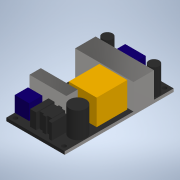
# Autodesk Inventor part: power unit
Saved by Autodesk Inventor 2022 (Build 260153000, 153)
## iProperties
Created: 2024-07-06
Part Number: power unit
Material: Типовые
Document SubType Name: Modeling
Designer: Капустяник Андрей
Density: 1 g/cm^3
Appearance: По умолчанию
Author: Капустяник Андрей
Autodesk Inventor part; units mm, degrees
ref_plane "YZ Plane" through (0, 0, 0) normal (1, 0, 0) x (0, 1, 0)
ref_plane "XZ Plane" through (0, 0, 0) normal (0, 1, 0) x (-1, 0, 0)
ref_plane "XY Plane" through (0, 0, 0) normal (0, 0, 1) x (1, 0, 0)
sketch "Эскиз1" plane through (0, 0, 0) normal (0, 1, 0) x (-1, 0, 0)
  line L0 (-28.51, 53.225) -> (28.51, 53.225)
  line L1 (28.51, 53.225) -> (28.51, -53.225)
  line L2 (28.51, -53.225) -> (-28.51, -53.225)
  line L3 (-28.51, -53.225) -> (-28.51, 53.225)
  line L4 (-28.51, 53.225) -> (28.51, -53.225) construction
  line L5 (28.51, 53.225) -> (-28.51, -53.225) construction
  line L6 (-23.7, 49.095) -> (23.7, 49.095)
  line L7 (23.7, 49.095) -> (23.7, -49.095)
  line L8 (23.7, -49.095) -> (-23.7, -49.095)
  line L9 (-23.7, -49.095) -> (-23.7, 49.095)
  line L10 (-23.7, 49.095) -> (23.7, -49.095) construction
  line L11 (23.7, 49.095) -> (-23.7, -49.095) construction
  circle A0 centre (23.7, 49.095) radius 2
  circle A1 centre (23.7, -49.095) radius 2
  circle A2 centre (-23.7, -49.095) radius 2
  circle A3 centre (-23.7, 49.095) radius 2
  point P0 (0, 0)
  dimension "d0" = 57.02
  dimension "d1" = 106.45
  dimension "d2" = 47.4
  dimension "d3" = 98.19
  dimension "d4" = 4
  dimension "d5" = 4
  dimension "d6" = 4
  dimension "d7" = 4
  constraints: 24 end point, 4 centre point, 4 coincident, 4 midpoint, 4 parallel, 2 horizontal, 2 perpendicular
  measures "d0" distance of L1.end L2.end
  measures "d1" distance of L0.end L1.end
  measures "d2" distance of L7.end L8.end
  measures "d3" distance of L6.end L7.end
  measures "d4" diameter of A0
  measures "d5" diameter of A1
  measures "d6" diameter of A2
  measures "d7" diameter of A3
extrude "Выдавливание1" add sketch "Эскиз1" along normal blind 28 contours L0 L1 L2 L3 | L6 A0 L7 A1 L8 A2 L9 A3
sketch "Эскиз2" plane through (0, 28, 0) normal (0, 1, 0) x (1, 0, 0)
  line L0 (-28.51, 53.225) -> (-28.51, -53.225) projected
  line L1 (-28.51, -53.225) -> (-28.51, 53.225) construction
  line L2 (-28.51, 53.225) -> (28.0416, 53.225) construction
  line L3 (28.0416, 53.225) -> (28.0416, -53.225) construction
  line L4 (28.0416, -53.225) -> (-28.51, -53.225) construction
  line L5 (-28.51, -53.225) -> (28.51, -53.225) projected
  line L6 (28.51, 53.225) -> (-28.51, 53.225) projected
  line L7 (28.51, -53.225) -> (28.51, 53.225) projected
  line L8 (-28.51, 14) -> (28.51, 14)
  line L9 (28.51, 14) -> (28.51, 34)
  line L10 (28.51, 34) -> (-28.51, 34)
  line L11 (-28.51, 34) -> (-28.51, 14)
  line L12 (-28.51, -30.6224) -> (7.5641, -30.6224)
  line L13 (7.5641, -30.6224) -> (7.5641, -19.5614)
  line L14 (7.5641, -19.5614) -> (-28.51, -19.5614)
  line L15 (-28.51, -19.5614) -> (-28.51, -30.6224)
  line L16 (-3.5371, -17.2143) -> (23.7214, -17.2143)
  line L17 (23.7214, -17.2143) -> (23.7214, 12.6792)
  line L18 (23.7214, 12.6792) -> (-3.5371, 12.6792)
  line L19 (-3.5371, 12.6792) -> (-3.5371, -17.2143)
  line L20 (-28.51, -45) -> (-14.5287, -45)
  line L21 (-14.5287, -45) -> (-14.5287, -32.0623)
  line L22 (-14.5287, -32.0623) -> (-28.51, -32.0623)
  line L23 (-28.51, -32.0623) -> (-28.51, -45)
  line L24 (-17.6681, 42.9169) -> (2.3645, 42.9169)
  line L25 (2.3645, 42.9169) -> (2.3645, 52.0693)
  line L26 (2.3645, 52.0693) -> (-17.6681, 52.0693)
  line L27 (-17.6681, 52.0693) -> (-17.6681, 42.9169)
  circle A0 centre (19.9269, -31.855) radius 8.0015
  line L28 (-9.1994, -49.3307) -> (-3.3498, -49.3307)
  line L29 (-3.3498, -49.3307) -> (-3.3498, -31.3319)
  line L30 (-3.3498, -31.3319) -> (-9.1994, -31.3319)
  line L31 (-9.1994, -31.3319) -> (-9.1994, -49.3307)
  line L32 (13.1822, -35.833) -> (9.6203, -35.833)
  line L33 (9.6203, -35.833) -> (9.6203, -49.5593)
  line L34 (10.6203, -50.5593) -> (13.1822, -50.5593)
  line L35 (13.1822, -50.5593) -> (13.1822, -35.833)
  line L36 (10.6203, -50.5593) -> (9.6203, -49.5593)
  line L37 (-2.5627, -46.539) -> (9.1983, -46.539)
  line L38 (9.1983, -46.539) -> (9.1983, -33.5613)
  line L39 (9.1983, -33.5613) -> (-2.5627, -33.5613)
  line L40 (-2.5627, -33.5613) -> (-2.5627, -46.539)
  line L41 (1.7463, -48.1105) -> (4.9907, -48.1105)
  line L42 (4.9907, -48.1105) -> (4.9907, -32.1926)
  line L43 (4.9907, -32.1926) -> (1.7463, -32.1926)
  line L44 (1.7463, -32.1926) -> (1.7463, -48.1105)
  circle A1 centre (-23, 40) radius 4.9506
  circle A2 centre (22.6723, 39.8615) radius 5.013
  point P0 (0, 0)
  point P1 (-28.51, 34)
  point P2 (28.51, 14)
  point P3 (9.6203, -50.5593)
  point P4 (4.9907, -46.539)
  point P5 (1.7463, -46.539)
  point P6 (1.7463, -33.5613)
  point P7 (4.9907, -33.5613)
  point P8 (12.9842, -35.833)
  point P9 (13.1822, -36.1601)
  dimension "d25" = 1
  dimension "d26" = 1
  constraints: 76 end point, 18 parallel, 9 horizontal, 9 perpendicular, 6 point on line, 3 centre point, 3 collinear, 2 other
  measures "d25" distance of L34.start point (9.62, -50.559)
  measures "d26" distance of L33.end point (9.62, -50.559)
extrude "Выдавливание2" cut sketch "Эскиз2" against normal blind 25 contours L6 L7 L10 L0 | L8 L7 L5 L0 L20 L21 L22 L12 L13 L14 | L32 L35 A0 picked at (13.1596, -36.015)
sketch "Эскиз3" plane through (0, 28, 0) normal (0, 1, 0) x (1, 0, 0)
  line L0 (-14.5287, -32.0623) -> (-28.51, -32.0623)
  line L1 (-28.51, -32.0623) -> (-28.51, -45)
  line L2 (-28.51, -45) -> (-14.5287, -45)
  line L3 (-14.5287, -45) -> (-14.5287, -32.0623)
  line L4 (2.3645, 52.0693) -> (-17.6681, 52.0693)
  line L5 (-17.6681, 52.0693) -> (-17.6681, 42.9169)
  line L6 (-17.6681, 42.9169) -> (2.3645, 42.9169)
  line L7 (2.3645, 42.9169) -> (2.3645, 52.0693)
  line L8 (4.9907, -46.539) -> (9.1983, -46.539)
  line L9 (9.1983, -46.539) -> (9.1983, -33.5613)
  line L10 (9.1983, -33.5613) -> (4.9907, -33.5613)
  line L11 (4.9907, -33.5613) -> (4.9907, -32.1926)
  line L12 (4.9907, -32.1926) -> (1.7463, -32.1926)
  line L13 (1.7463, -32.1926) -> (1.7463, -33.5613)
  line L14 (1.7463, -33.5613) -> (-2.5627, -33.5613)
  line L15 (-2.5627, -33.5613) -> (-2.5627, -46.539)
  line L16 (-2.5627, -46.539) -> (1.7463, -46.539)
  line L17 (1.7463, -46.539) -> (1.7463, -48.1105)
  line L18 (1.7463, -48.1105) -> (4.9907, -48.1105)
  line L19 (4.9907, -48.1105) -> (4.9907, -46.539)
  line L20 (-3.3498, -31.3319) -> (-9.1994, -31.3319)
  line L21 (-9.1994, -31.3319) -> (-9.1994, -49.3307)
  line L22 (-9.1994, -49.3307) -> (-3.3498, -49.3307)
  line L23 (-3.3498, -49.3307) -> (-3.3498, -31.3319)
  line L24 (12.9842, -35.833) -> (9.6203, -35.833)
  line L25 (9.6203, -35.833) -> (9.6203, -49.5593)
  line L26 (9.6203, -49.5593) -> (10.6203, -50.5593)
  line L27 (10.6203, -50.5593) -> (13.1822, -50.5593)
  line L28 (13.1822, -50.5593) -> (13.1822, -36.1601)
  arc A0 (13.1822, -36.1601) -> (12.9842, -35.833) centre (19.9269, -31.855) ccw
  line L29 (12.9842, -35.833) -> (13.1822, -35.833)
  line L30 (13.1822, -35.833) -> (13.1822, -36.1601)
  arc A1 (12.9842, -35.833) -> (13.1822, -36.1601) centre (19.9269, -31.855) ccw
  circle A2 centre (-23, 40) radius 4.9506
  circle A3 centre (22.6723, 39.8615) radius 5.013
  point P0 (0, 0)
extrude "Выдавливание3" cut sketch "Эскиз3" against normal blind 10 contours L3 L2 L1 L0 | L7 L6 L5 L4 | L19 L18 L17 L16 L15 L14 L13 L12 L11 L10 L9 L8 | L23 L22 L21 L20 | A1 L28 L27 L26 L25 L24
equation "\"d26\" = d25"
